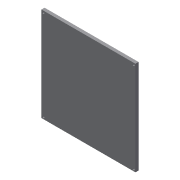
# Autodesk Inventor part: aanstuurkast kap
Saved by Autodesk Inventor 2019 (Build 230136000, 136)
## iProperties
Created: 2020-02-29
Part Number: aanstuurkast kap
Material: Generic
Document SubType Name: Modeling
Designer: stef_
Density: 1 g/cm^3
Appearance: Default
Author: stef_
Autodesk Inventor part; units mm, degrees
ref_plane "YZ Plane" through (0, 0, 0) normal (1, 0, 0) x (0, 1, 0)
ref_plane "XZ Plane" through (0, 0, 0) normal (0, 1, 0) x (-1, 0, 0)
ref_plane "XY Plane" through (0, 0, 0) normal (0, 0, 1) x (1, 0, 0)
sketch "Sketch1" plane through (0, 0, 0) normal (0, 0, 1) x (1, 0, 0)
  circle A0 centre (144, -144) radius 3.3235 projected
  circle A1 centre (-144, 144) radius 3.3235 projected
  circle A2 centre (144, 144) radius 3.3235 projected
  circle A3 centre (-144, -144) radius 3.3235 projected
  line L0 (140, 140) -> (140, -140) projected
  line L1 (140, -140) -> (-140, -140) projected
  line L2 (-140, -140) -> (-140, 140) projected
  line L3 (-140, 140) -> (140, 140) projected
  line L4 (150, 150) -> (-150, 150) projected
  line L5 (-150, 150) -> (-150, -150) projected
  line L6 (-150, -150) -> (150, -150) projected
  line L7 (150, -150) -> (150, 150) projected
  line L8 (-150, 150) -> (150, 150)
  line L9 (150, 150) -> (150, -150)
  line L10 (150, -150) -> (-150, -150)
  line L11 (-150, -150) -> (-150, 150)
  circle A4 centre (-144, 144) radius 3.3235
  circle A5 centre (144, 144) radius 3.3235
  circle A6 centre (144, -144) radius 3.3235
  circle A7 centre (-144, -144) radius 3.3235
  point P0 (0, 0)
  constraints: 8 end point, 4 centre point, 4 coincident, 4 concentric, 2 parallel, 1 horizontal, 1 perpendicular
extrude "Extrusion1" add sketch "Sketch1" along normal blind 10 contours L0 L1 L2 L3 | L7 L6 L5 L4
body "Solid1"
